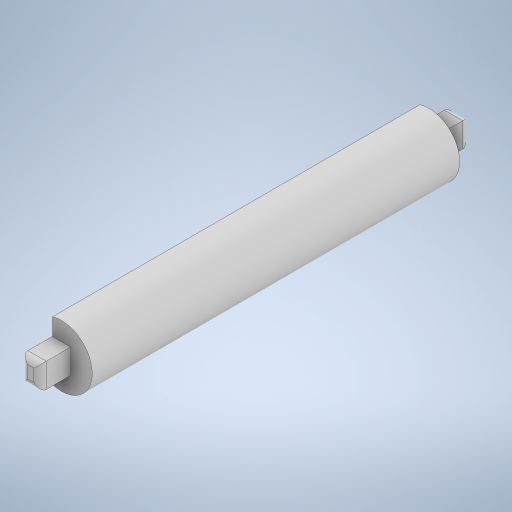
# Autodesk Inventor part: 茎固定パーツ2
Saved by Autodesk Inventor 2024.3 (Build 283343000, 343)
## iProperties
Created: 2024-10-08
Part Number: 茎固定パーツ2
Material: 一般
Document SubType Name: Modeling
Designer: hikou
Density: 1 g/cm^3
Appearance: 既定
Author: hikou
Autodesk Inventor part; units mm, degrees
ref_plane "YZ Plane" through (0, 0, 0) normal (1, 0, 0) x (0, 1, 0)
ref_plane "XZ Plane" through (0, 0, 0) normal (0, 1, 0) x (-1, 0, 0)
ref_plane "XY Plane" through (0, 0, 0) normal (0, 0, 1) x (1, 0, 0)
sketch "スケッチ1" plane through (0, 0, 0) normal (0, 0, 1) x (1, 0, 0)
  circle A0 centre (0, 0) radius 5
  dimension "d0" = 10
  constraints: 1 centre point, 1 coincident
  measures "d0" diameter of A0
extrude "押し出し1" add sketch "スケッチ1" along normal mid plane 60
sketch "スケッチ2" plane through (0, 0, 30) normal (0, 0, 1) x (1, 0, 0)
  line L0 (-1.5, -2) -> (1.5, -2)
  line L1 (1.5, -2) -> (1.5, 2)
  line L2 (1.5, 2) -> (-1.5, 2)
  line L3 (-1.5, 2) -> (-1.5, -2)
  line L4 (-1.5, -2) -> (1.5, 2) construction
  line L5 (1.5, -2) -> (-1.5, 2) construction
  point P0 (0, 0)
  dimension "d3" = 3
  dimension "d4" = 4
  constraints: 12 end point, 2 midpoint, 2 parallel, 1 horizontal, 1 perpendicular
  measures "d3" distance of L2.end L1.end
  measures "d4" distance of L0.end L1.end
extrude "押し出し2" add sketch "スケッチ2" along normal blind 5
sketch "スケッチ3" plane through (0, 0, -30) normal (0, 0, -1) x (-1, 0, 0)
  line L0 (1.5, -2) -> (1.5, 2) projected
  line L1 (1.5, 2) -> (-1.5, 2) projected
  line L2 (-1.5, -2) -> (1.5, -2) projected
  line L3 (-1.5, 2) -> (-1.5, -2) projected
  point P0 (0, 0)
extrude "押し出し3" add sketch "スケッチ3" along normal blind 5
fillet "フィレット1" radius 1 8 edges at (-1.5, 0, -35) (0, 2, -35) (0, -2, -35) (1.5, 0, -35) (-1.5, 0, 35) (0, 2, 35) (1.5, 0, 35) (0, -2, 35)
sketch "スケッチ4" plane through (0, 0, 30) normal (0, 0, 1) x (1, 0, 0)
  line L0 (1.5, -2) -> (-1.5, -2) projected
  line L1 (-1.5, -2) -> (-1.5, 2) projected
  line L2 (-1.5, 2) -> (1.5, 2) projected
  line L3 (1.5, 2) -> (1.5, -2) projected
  circle A0 centre (0, 0) radius 5 projected
  line L4 (-1.5, 2) -> (-1.5, -2) projected
  line L5 (-1.5, 2) -> (-1.5, -2) projected
  line L6 (-1.5, 2) -> (-1.5, 4.7697)
  line L7 (-1.5, -2) -> (-1.5, -4.7697)
  constraints: 4 end point, 2 point on circle, 2 point on line
extrude "押し出し4" cut sketch "スケッチ4" against normal through all contours L7 A0 L6 L1
